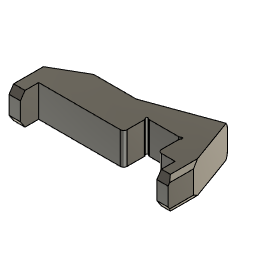
Z Linear Rail Jig v5 (Autodesk Fusion 360 design; units mm, degrees)
Autodesk Fusion 360 part; units mm, degrees
sketch "Sketch1" plane through (0, 0, 0) normal (0, 0, 1) x (1, 0, 0)
  line L0 (0, 0) -> (0, 8)
  line L1 (0, 8) -> (37.45, 8)
  line L2 (37.45, 8) -> (37.45, 18.2)
  line L3 (37.45, 18.2) -> (52.55, 18.2)
  line L4 (52.55, 18.2) -> (52.55, 8)
  line L5 (52.55, 8) -> (60.05, 8)
  line L6 (60.05, 8) -> (60.05, 0)
  line L7 (60.05, 0) -> (65, 0)
  line L8 (65, 0) -> (65, 11.2)
  line L9 (24.8746, 23.2) -> (-5, 23.2)
  line L10 (-5, 23.2) -> (-5, 0)
  line L11 (-5, 0) -> (0, 0)
  line L12 (65, 11.2) -> (56.4495, 34.6923)
  line L13 (24.8746, 23.2) -> (56.4495, 34.6923)
  dimension "d4" = 10.2
  dimension "d5" = 15.1
  dimension "d6" = 5
  dimension "d7" = 5
  dimension "d8" = 8
  dimension "d26" = 70
  dimension "d27" = 60.05
  dimension "d28" = 7.5
  dimension "d30" = 20
  dimension "d31" = 12
  dimension "d32" = 90
  dimension "d33" = 25
  constraint coincident L0.start L11.end
  constraint vertical L0
  constraint perpendicular L0 L1
  constraint perpendicular L1 L2
  constraint perpendicular L2 L3
  constraint perpendicular L3 L4
  constraint perpendicular L4 L5
  constraint collinear L1 L5
  constraint perpendicular L5 L6
  constraint perpendicular L6 L7
  constraint perpendicular L7 L8
  constraint perpendicular L6 L9
  constraint perpendicular L9 L10
  constraint perpendicular L0 L11
  constraint collinear L7 L11
  measures "d4" distance of L1.end L2.end
  measures "d5" distance of L2.end L3.end
  measures "d6" distance of L0 L10
  measures "d7" distance of L3 L9
  measures "d8" distance of L1 L11
  measures "d26" distance of L8 L10
  measures "d27" distance of L0 L6
  measures "d28" distance of L4.end L5.end
  measures "d30" angle of L8 L12
  measures "d31" distance of L9 L8.end
  measures "d32" angle of L12 L13
  measures "d33" distance of L8.end L13
extrude "Extrude1" add sketch "Sketch1" along normal blind 14
chamfer "Chamfer1" distance 12 angle 30 1 edges at (-5, 23.2, 7) measured on face at (14.9164, 23.2, 4.6667)
fillet "Fillet1" radius 1.5 2 edges at (37.45, 8, 7) (52.55, 8, 7)
sketch "Sketch2" plane through (0, 0, 14) normal (0, 0, 1) x (-1, 0, 0)
  arc A0 (-52.55, -9.5) -> (-54.05, -8) centre (-54.05, -9.5) ccw
  line L0 (-54.05, -8) -> (-60.05, -8)
  line L1 (-60.05, -8) -> (-60.05, 0)
  line L2 (-60.05, 0) -> (-65, 0)
  line L3 (-65, 0) -> (-65, -11.2)
  line L4 (-24.8746, -23.2) -> (-7, -23.2)
  line L5 (-7, -23.2) -> (5, -16.2718)
  line L6 (5, -16.2718) -> (5, 0)
  line L7 (5, 0) -> (0, 0)
  line L8 (0, 0) -> (0, -8)
  line L9 (0, -8) -> (-35.95, -8)
  arc A1 (-35.95, -8) -> (-37.45, -9.5) centre (-35.95, -9.5) ccw
  line L10 (-37.45, -9.5) -> (-37.45, -18.2)
  line L11 (-37.45, -18.2) -> (-52.55, -18.2)
  line L12 (-52.55, -18.2) -> (-52.55, -9.5)
  circle A2 centre (-37.45, -18.2) radius 0.5
  circle A3 centre (-52.55, -18.2) radius 0.5
  line L13 (-65, -11.2) -> (-56.4495, -34.6923)
  line L14 (-56.4495, -34.6923) -> (-24.8746, -23.2)
  dimension "d16" = 1
  constraint coincident L10.end L11.start
  constraint coincident L11.end L12.start
  constraint equal A2 A3
  measures "d16" diameter of A3
extrude "Extrude2" cut sketch "Sketch2" against normal through all contours L11 L12 A3 | L10 L11 A2 picked at (-52.5418, -18.5323) picked at (-37.7815, -18.2248)
fillet "Fillet2" radius 1 4 edges at (37.45, 17.7, 7) (37.95, 18.2, 7) (52.05, 18.2, 7) (52.55, 17.7, 7)
chamfer "Chamfer2" distance 2 distance2 1 3 edges at (1, 19.7359, 14) (1, 19.7359, 0) (65, 5.6, 0) measured on face at (-1, 18.5812, 4.6667) measured on face at (-1, 18.5812, 4.6667) measured on face at (65, 3.7333, 4.6667)
chamfer "Chamfer2" distance 1 distance2 2 3 edges at (65, 5.6, 14) (40.6621, 28.9462, 14) (40.6621, 28.9462, 0) measured on face at (20.2749, 13.0667, 14) measured on face at (20.2749, 13.0667, 14) measured on face at (20.2749, 13.0667, 0)
chamfer "Chamfer3" distance 2 distance2 3 2 edges at (62.525, 0, 14) (-2.5, 0, 14) measured on face at (14.9833, 13.0667, 14) measured on face at (14.9833, 13.0667, 14)
chamfer "Chamfer3" distance 3 distance2 2 2 edges at (62.525, 0, 0) (-2.5, 0, 0) measured on face at (61.7, 0, 8.6667) measured on face at (-3.3333, 0, 4.6667)
